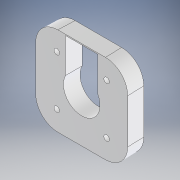
# Autodesk Inventor part: AA035
Saved by Autodesk Inventor 2017 SP1 (Build 210196100, 196)
## iProperties
Created: 2017-10-23
Part Number: AA035
Material: ABS Plastic
Document SubType Name: Modeling
Designer: Zach
Categories: <?xml version="1.0" encoding="UTF-16"?> <MemberInstance><Categories><FamilyTemplate><FamilyTemplateParameter ValueType="xs:double" Id="1" ObjectReferenceKey="da_z" ObjectType="kUserParameterObject"/><FamilyTemplateParameter ValueType="xs:double" Id="2" ObjectReferenceKey="da_b" ObjectType="kUserParameterObject"/><FamilyTemplateParameter ValueType="xs:double" Id="3" ObjectReferenceKey="da_beta" ObjectType="kUserParameterObject"/><FamilyTemplateParameter ValueType="xs:double" Id="4" ObjectReferenceKey="da_da" ObjectType="kUserParameterObject"/><FamilyTemplateParameter ValueType="xs:double" Id="5" ObjectReferenceKey="da_aw" ObjectType="kUserParameterObject"/><FamilyTemplateParameter ValueType="xs:string" Id="6" ObjectReferenceKey="EAIAABAAAACIAQAAAAAAAIAAAAAAAAAA" ObjectType="83910656" SubObjectId="SurfaceGeometry"/></FamilyTemplate><ParamToTemplateMap><ParamToTemplate CategoryParameter="//CategoryParameter[@InternalName='046C89C9-8512-4d59-83FE-43B91F4F132A']" TemplateParameter="1"/><ParamToTemplate CategoryParameter="//CategoryParameter[@InternalName='2552DF32-E462-4b46-AEBF-C6C7768E72AC']" TemplateParameter="2"/><ParamToTemplate CategoryParameter="//CategoryParameter[@InternalName='C9EE641D-15FC-4fae-A226-E94C4372FDD7']" TemplateParameter="3"/><ParamToTemplate><ParamToTemplate CategoryParameter="//CategoryParameter[@InternalName='00B6519A-459B-49c7-AD84-2E56D39A5744']" ConstantValue="0.341447"/></ParamToTemplate><ParamToTemplate><ParamToTemplate CategoryParameter="//CategoryParameter[@InternalName='04B31F0E-C7A6-4894-AA32-9629BEFACF47']" ConstantValue="1.000000"/></ParamToTemplate><ParamToTemplate><ParamToTemplate CategoryParameter="//CategoryParameter[@InternalName='43CBEC2E-7847-49e7-A936-2F7889FCB2D9']" ConstantValue="0.250000"/></ParamToTemplate><ParamToTemplate><ParamToTemplate CategoryParameter="//CategoryParameter[@InternalName='B1EFC894-105D-4ebd-86BF-FA20ED196853']" ConstantValue="0.350000"/></ParamToTemplate><ParamToTemplate><ParamToTemplate CategoryParameter="//CategoryParameter[@InternalName='51175063-3D10-4879-93E8-6246FE8B403D']" ConstantValue="2060000000.000000"/></ParamToTemplate><ParamToTemplate><ParamToTemplate CategoryParameter="//CategoryParameter[@InternalName='A3A52E27-4454-46a9-B0BD-C932399B70AF']" ConstantValue="0.300000"/></ParamToTemplate><ParamToTemplate><ParamToTemplate CategoryParameter="//CategoryParameter[@InternalName='91B76062-C214-41d9-B1B9-14D2AB99603D']" ConstantValue="0.200000"/></ParamToTemplate><ParamToTemplate><ParamToTemplate CategoryParameter="//CategoryParameter[@InternalName='374E806E-8B8A-4dda-A9AA-1039D6500AD2']" ConstantValue="5.000000"/></ParamToTemplate><ParamToTemplate><ParamToTemplate CategoryParameter="//CategoryParameter[@InternalName='2D373A89-B862-43d6-8D0B-0CBF12AB9F6C']" ConstantValue="0.392699"/></ParamToTemplate><ParamToTemplate CategoryParameter="//CategoryParameter[@InternalName='37777632-D6A2-4fac-9D53-DB8ACD95C989']" TemplateParameter="4"/><ParamToTemplate CategoryParameter="//CategoryParameter[@InternalName='FD1017F1-B727-4f7e-9707-0F86F1FF9423']" TemplateParameter="5"/><ParamToTemplate><ParamToTemplate CategoryParameter="//CategoryParameter[@InternalName='9E1B4470-B2D3-4ff1-B813-535BB4CDF51A']" ConstantValue="3520000.000000"/></ParamToTemplate><ParamToTemplate><ParamToTemplate CategoryParameter="//CategoryParameter[@InternalName='F8452263-BFF6-458c-9FB1-07C4B99E95CD']" ConstantValue="11400000.000000"/></ParamToTemplate><ParamToTemplate><ParamToTemplate CategoryParameter="//CategoryParameter[@InternalName='3E3BB259-FD49-497f-8171-6EBC954A3479']" ConstantValue="2.000000"/></ParamToTemplate><ParamToTemplate CategoryParameter="//CategoryParameter[@InternalName='27C3BAF2-7550-4e4b-AE2C-0DB134B7D9B7']" TemplateParameter="6"/></ParamToTemplateMap><Category DisplayName="Gear" InternalName="DC85795E-93AB-48d5-8EEE-5A27447B64BD" Mnemonic="Gear"><CategoryParameter DisplayName="z" InternalName="046C89C9-8512-4d59-83FE-43B91F4F132A" Mnemonic="z"/><CategoryParameter DisplayName="b" InternalName="2552DF32-E462-4b46-AEBF-C6C7768E72AC" Mnemonic="b"/><CategoryParameter DisplayName="||b|" InternalName="C9EE641D-15FC-4fae-A226-E94C4372FDD7" Mnemonic="beta"/><CategoryParameter DisplayName="x" InternalName="00B6519A-459B-49c7-AD84-2E56D39A5744" Mnemonic="x"/><CategoryParameter DisplayName="a*" InternalName="04B31F0E-C7A6-4894-AA32-9629BEFACF47" Mnemonic="a"/><CategoryParameter DisplayName="c*" InternalName="43CBEC2E-7847-49e7-A936-2F7889FCB2D9" Mnemonic="c"/><CategoryParameter DisplayName="r|.f|*" InternalName="B1EFC894-105D-4ebd-86BF-FA20ED196853" Mnemonic="rf"/><CategoryParameter DisplayName="E" InternalName="51175063-3D10-4879-93E8-6246FE8B403D" Mnemonic="E"/><CategoryParameter DisplayName="||m|" InternalName="A3A52E27-4454-46a9-B0BD-C932399B70AF" Mnemonic="mi"/><Category DisplayName="SpurGear" InternalName="26C5A22E-A91E-4dfd-A3B3-23CCAFAE1764" Mnemonic="SpurGear"><CategoryParameter DisplayName="m" InternalName="91B76062-C214-41d9-B1B9-14D2AB99603D" Mnemonic="m"/><CategoryParameter DisplayName="P" InternalName="374E806E-8B8A-4dda-A9AA-1039D6500AD2" Mnemonic="PP"/><CategoryParameter DisplayName="||a|" InternalName="2D373A89-B862-43d6-8D0B-0CBF12AB9F6C" Mnemonic="alpha"/><CategoryParameter DisplayName="d|.a|" InternalName="37777632-D6A2-4fac-9D53-DB8ACD95C989" Mnemonic="da"/><CategoryParameter DisplayName="a|.w|" InternalName="FD1017F1-B727-4f7e-9707-0F86F1FF9423" Mnemonic="aw"/><CategoryParameter DisplayName="||s||.Flim|" InternalName="9E1B4470-B2D3-4ff1-B813-535BB4CDF51A" Mnemonic="sFlim"/><CategoryParameter DisplayName="||s||.Hlim|" InternalName="F8452263-BFF6-458c-9FB1-07C4B99E95CD" Mnemonic="sHlim"/><CategoryParameter DisplayName="type" InternalName="3E3BB259-FD49-497f-8171-6EBC954A3479" Mnemonic="type"/><CategoryParameter DisplayName="PitchDiameter" InternalName="27C3BAF2-7550-4e4b-AE2C-0DB134B7D9B7" Mnemonic="IDS_PITCHDIAM"/></Category></Category></Categories></MemberInstance>
Density: 1.06 g/cm^3
Appearance: CR White
CustomPartVersion: 1
Author: Zach
Autodesk Inventor part; units mm, degrees
ref_plane "YZ Plane" through (0, 0, 0) normal (1, 0, 0) x (0, 1, 0)
ref_plane "XZ Plane" through (0, 0, 0) normal (0, 1, 0) x (-1, 0, 0)
ref_plane "XY Plane" through (0, 0, 0) normal (0, 0, 1) x (1, 0, 0)
sketch "Sketch3" plane through (0, 0, 0) normal (0, 0, 1) x (1, 0, 0)
  circle A0 centre (0, 0) radius 60
  dimension "d49" = 120
  constraints: 1 centre point, 1 coincident
  measures "d49" diameter of A0
extrude "Extrusion2" add sketch "Sketch3" along normal blind 67
sketch "Sketch4" plane through (0, 0, 0) normal (0, 0, -1) x (-1, 0, 0)
  circle A0 centre (0, 0) radius 4.25
  dimension "d52" = 8.5
  constraints: 1 centre point, 1 coincident
  measures "d52" diameter of A0
extrude "Extrusion3" cut sketch "Sketch4" against normal through all
ref_plane "Work Plane11" through (0, 0, 46) normal (0, 0, 1) x (1, 0, 0)
sketch "Sketch6" plane through (0, 0, 46) normal (0, 0, 1) x (1, 0, 0)
  line L0 (-27.5, -53.3268) -> (27.5, -53.3268)
  line L1 (27.5, -53.3268) -> (27.5, -61.3268)
  line L2 (27.5, -61.3268) -> (-27.5, -61.3268)
  line L3 (-27.5, -61.3268) -> (-27.5, -53.3268)
  circle A0 centre (0, 0) radius 4.25 construction
  circle A1 centre (0, 0) radius 60 construction
  dimension "d63" = 55
  dimension "d64" = 8
  constraints: 8 end point, 2 parallel, 2 point on circle, 1 horizontal, 1 perpendicular
  measures "d63" distance of L1.end L2.end
  measures "d64" distance of L0.end L1.end
extrude "Extrusion5" add sketch "Sketch6" along normal mid plane 42
sketch "Sketch7" plane through (0, 0, 46) normal (0, 0, 1) x (1, 0, 0)
  line L0 (-41, -61.3268) -> (41, -61.3268)
  line L1 (41.5215, -76.3268) -> (-41.5215, -76.3268)
  line L2 (27.5, -61.3268) -> (-27.5, -61.3268) projected
  line L3 (-41.5215, -76.3268) -> (-41, -61.3268)
  line L4 (41.5215, -76.3268) -> (41, -61.3268)
  point P0 (0, 0)
  point P1 (0, -61.3268)
  point P2 (0, -76.3268)
  dimension "d67" = 83.043
  dimension "d99" = 82
  dimension "d100" = 15
  constraints: 8 end point, 3 midpoint, 1 horizontal, 1 parallel, 1 vertical alignment
  measures "d67" distance of L1.start L1.end
  measures "d99" distance of L0.start L0.end
  measures "d100" distance between parallel lines of L0 L1
extrude "Extrusion6" add sketch "Sketch7" along normal mid plane 80
sketch "Sketch8" plane through (-41.5215, -76.3268, 86) normal (0, -1, 0) x (1, 0, 0)
  line L0 (64.0215, -62.5) -> (19.0215, -62.5) construction
  line L1 (19.0215, -62.5) -> (19.0215, -17.5) construction
  line L2 (19.0215, -17.5) -> (64.0215, -17.5) construction
  line L3 (64.0215, -17.5) -> (64.0215, -62.5) construction
  circle A0 centre (64.0215, -62.5) radius 2.5
  circle A1 centre (64.0215, -17.5) radius 2.5
  circle A2 centre (19.0215, -62.5) radius 2.5
  circle A3 centre (19.0215, -17.5) radius 2.5
  line L4 (0, 0) -> (83.043, 0) projected
  line L5 (83.043, 0) -> (83.043, -80) projected
  point P0 (23.25, -86)
  point P1 (41.5215, -17.5)
  point P2 (41.5215, 0)
  point P3 (64.0215, -40)
  point P4 (83.043, -40)
  dimension "d75" = 45
  dimension "d78" = 5
  dimension "d79" = 5
  dimension "d101" = 45
  dimension "d102" = 5
  dimension "d103" = 5
  constraints: 8 end point, 4 centre point, 4 coincident, 4 midpoint, 2 parallel, 1 horizontal, 1 horizontal alignment, 1 perpendicular, 1 vertical alignment
  measures "d75" distance of L0.end L1.end
  measures "d78" diameter of A2
  measures "d79" diameter of A3
  measures "d101" distance of L1.end L2.end
  measures "d102" diameter of A1
  measures "d103" diameter of A0
extrude "Extrusion7" cut sketch "Sketch8" against normal blind 25
sketch "Sketch9" plane through (-41.5215, -76.3268, 86) normal (0, -1, 0) x (1, 0, 0)
  circle A0 centre (41.5215, -40) radius 16.5
  circle A1 centre (19.0215, -62.5) radius 2.5 construction
  circle A2 centre (64.0215, -62.5) radius 2.5 construction
  circle A3 centre (64.0215, -17.5) radius 2.5 construction
  circle A4 centre (19.0215, -17.5) radius 2.5 construction
  line L0 (83.043, 0) -> (83.043, -80) construction
  line L1 (0, 0) -> (83.043, 0) construction
  line L2 (0, 0) -> (0, -80) construction
  line L3 (83.043, -80) -> (0, -80) construction
  point P0 (23.25, -86)
  point P1 (0, -40)
  point P2 (41.5215, 0)
  dimension "d82" = 33
  constraints: 2 midpoint, 1 centre point, 1 horizontal alignment, 1 vertical alignment
  measures "d82" diameter of A0
extrude "Extrusion8" cut sketch "Sketch9" against normal blind 45
sketch "Sketch14" plane through (0, 0, 46) normal (0, 0, 1) x (1, 0, 0)
  line L0 (16.5, -76.3268) -> (16.5, -31.3268) projected
  line L1 (16.5, -31.3268) -> (-16.5, -31.3268)
  line L2 (-16.5, -31.3268) -> (-16.5, -16.3268)
  line L3 (-16.5, -16.3268) -> (16.5, -16.3268)
  line L4 (16.5, -16.3268) -> (16.5, -31.3268)
  point P0 (0, 0)
  dimension "d91" = 33
  dimension "d92" = 15
  constraints: 8 end point, 2 parallel, 1 horizontal, 1 perpendicular
  measures "d91" distance of L2.end L3.end
  measures "d92" distance of L1.end L2.end
extrude "Extrusion10" cut sketch "Sketch14" along normal mid plane 33
sketch "Sketch15" plane through (16.5, -31.3268, 29.5) normal (-1, 0, 0) x (0, 0, 1)
  line L0 (33, 15) -> (0, 15) projected
  line L1 (0, 15) -> (0, 0) projected
  line L2 (0, 0) -> (16.5, 0) projected
  line L3 (16.5, 0) -> (33, 0) projected
  line L4 (33, 0) -> (33, 15) projected
  line L5 (24, 14) -> (9, 14)
  line L6 (9, 14) -> (9, 1)
  line L7 (9, 1) -> (24, 1)
  line L8 (24, 1) -> (24, 14)
  point P0 (-29.5, 31.3268)
  point P1 (16.5, 1)
  point P2 (24, 7.5)
  point P3 (33, 7.5)
  dimension "d95" = 15
  dimension "d96" = 13
  constraints: 8 end point, 3 midpoint, 2 parallel, 1 horizontal, 1 horizontal alignment, 1 perpendicular, 1 vertical alignment
  measures "d95" distance of L7.end L6.end
  measures "d96" distance of L6.end L5.end
extrude "Extrusion11" cut sketch "Sketch15" along normal through all contours L8 L7 L6 L5
fillet "Fillet4" radius 20 4 edges at (41.2608, -68.8268, 86) (41.2608, -68.8268, 6) (-41.2608, -68.8268, 86) (-41.2608, -68.8268, 6)
ref_plane "Work Plane15" through (0, 0, 25) normal (0, 0, -1) x (-0.9685832, -0.2486899, 0)
sketch "Sketch16" plane through (0, 0, 25) normal (0, 0, -1) x (-0.9685832, -0.2486899, 0)
  circle A0 centre (0, 0) radius 60
  circle A1 centre (0, 0) radius 63
  dimension "d107" = 3
  constraints: 2 centre point
  measures "d107" radial gap between concentric circles of A0 A1
extrude "Extrusion12" cut sketch "Sketch16" along normal through all contours A0 | A1
sketch "Sketch17" plane through (0, 0, 25) normal (0, 0, -1) x (-1, 0, 0)
  circle A0 centre (33.9004, 8.7041) radius 2.5
  circle A1 centre (9.4122, 33.7107) radius 2.5
  circle A2 centre (-24.4882, 25.0065) radius 2.5
  circle A3 centre (-33.9004, -8.7041) radius 2.5
  circle A4 centre (-9.4122, -33.7107) radius 2.5
  circle A5 centre (24.4882, -25.0065) radius 2.5
  line L0 (33.9004, 8.7041) -> (-33.9004, -8.7041) construction
  line L1 (-1.7981, -79.488) -> (39.8693, -68.7896)
  point P0 (0, 0)
  dimension "d108" = 5
  dimension "d109" = 35
  dimension "d112" = 360
  constraints: 6 centre point, 4 end point, 1 parallel, 13 other
  measures "d108" diameter of A0
  measures "d109" distance of point (0, 0) L0.start
extrude "Extrusion13" cut sketch "Sketch17" against normal blind 25 contours A0 | A1 | A2 | A3
sketch "Sketch20" plane through (0, 0, 67) normal (0, 0, 1) x (1, 0, 0)
  arc A0 (27.5, -53.3268) -> (-27.5, -53.3268) centre (0, 0) ccw projected
  circle A1 centre (0, 0) radius 60
  circle A2 centre (0, 0) radius 4.25 projected
  constraints: 1 coincident, 3 other
extrude "Extrusion15" add sketch "Sketch20" along normal blind 25
sketch "Sketch21" plane through (-21.5094, -76.3268, 6) normal (0, -1, 0) x (1, 0, 0)
  line L0 (36.0094, 79) -> (7.0094, 79)
  line L1 (7.0094, 79) -> (7.0094, 55)
  line L2 (7.0094, 55) -> (36.0094, 55)
  line L3 (36.0094, 55) -> (36.0094, 79)
  circle A0 centre (21.5094, 40) radius 16.5 projected
  line L4 (36.0094, 67) -> (7.0094, 67)
  point P0 (21.5094, -6)
  point P1 (21.5094, 67)
  dimension "d124" = 29
  dimension "d125" = 24
  dimension "d126" = 27
  constraints: 10 end point, 3 midpoint, 2 parallel, 1 horizontal, 1 perpendicular, 1 vertical alignment
  measures "d124" distance of L2.end L1.end
  measures "d125" distance of L1.end L0.end
  measures "d126" distance from line of L4 A0.centre
extrude "Extrusion16" cut sketch "Sketch21" against normal blind 15 contours L3 L4 L1 L0 | L3 L2 A0 L1 L4 | L2 A0 picked at (22.682, 55.3735)
sketch "Sketch22" plane through (-27.5, -61.3268, 67) normal (0, 1, 0) x (1, 0, 0)
  line L0 (55, 0) -> (55, 42) projected
  line L1 (0, 0) -> (0, 42) projected
  line L2 (0, 0) -> (3, 0)
  line L3 (55, 0) -> (55, -17.9115)
  line L4 (0, 0) -> (0, -17.9115)
  line L5 (5.9906, -19) -> (6.5121, -19) construction
  line L6 (-13.5, 1) -> (-14.0215, 1) construction
  circle A0 centre (5, -1.5) radius 2.5 projected
  line L7 (42, -18) -> (42, 6) projected
  line L8 (13, -18) -> (42, -18) projected
  line L9 (13, 6) -> (13, -18) projected
  line L10 (7, 0) -> (13, 0)
  line L11 (13, 0) -> (13, -18)
  line L12 (13, -18) -> (42, -18)
  line L13 (55, 0) -> (52, 0)
  circle A1 centre (50, -1.5) radius 2.5 projected
  line L14 (48, 0) -> (42, 0)
  line L15 (42, 0) -> (42, -18)
  arc A2 (48, 0) -> (52, 0) centre (50, -1.5) ccw
  arc A3 (3, 0) -> (7, 0) centre (5, -1.5) ccw
  line L16 (5.9906, -19) -> (6.2858, -19) projected
  line L17 (-13.5, 1) -> (-14.0215, 1) projected
  line L18 (5.9906, -19) -> (6.5121, -19) projected
  line L19 (48.4879, -19) -> (49.0094, -19) projected
  arc A4 (0, -17.9115) -> (6.2858, -19) centre (6.5121, 1) ccw
  arc A5 (48.4879, -19) -> (55, -17.9115) centre (48.488, 1.023) ccw
  line L20 (48.4879, -19) -> (6.2858, -19)
  line L21 (5.9906, -19) -> (49.0094, -19) projected
  ellipse E0 centre (5.9906, 1) end of major axis (-14.0215, 1) minor radius 20 (-14.0215, 1) -> (5.9906, -19) ccw projected
  line L22 (5.9906, -19) -> (6.5121, -19) projected
  ellipse E1 centre (6.5121, 1) end of major axis (-13.5, 1) minor radius 20 (-13.5, 1) -> (6.5121, -19) ccw projected
  line L23 (-13.5, 1) -> (-14.0215, 1) projected
  ellipse E2 centre (48.4879, 1) end of major axis (68.5, 1) minor radius 20 (48.4879, -19) -> (68.5, 1) ccw projected
  line L24 (48.4879, -19) -> (49.0094, -19) projected
  ellipse E3 centre (49.0094, 1) end of major axis (69.0215, 1) minor radius 20 (49.0094, -19) -> (69.0215, 1) ccw projected
  line L25 (69.0215, 1) -> (68.5, 1) projected
  point P0 (27.5, 67)
  point P1 (51.7891, -18.726)
  constraints: 22 end point, 11 point on circle, 4 centre point, 4 point on line, 3 perpendicular, 2 coincident, 2 collinear, 2 vertical, 1 horizontal, 1 horizontal alignment, 10 other
extrude "Extrusion17" add sketch "Sketch22" along normal blind 15 contours L2 A0 L10 L9 L8 L7 L14 A1 L13 L3 A5 L20 L18 A4 L4
sketch "Sketch23" plane through (-21.5094, -76.3268, 6) normal (0, -1, 0) x (1, 0, 0)
  line L0 (36.0094, 79) -> (36.0094, 55) projected
  line L1 (36.0094, 55) -> (7.0094, 55) projected
  line L2 (7.0094, 55) -> (7.0094, 79) projected
  line L3 (7.0094, 79) -> (36.0094, 79) projected
  point P0 (21.5094, -6)
extrude "Extrusion18" cut sketch "Sketch23" against normal blind 20
sketch "Sketch25" plane through (-21.5094, -56.3268, 6) normal (0, -1, 0) x (1, 0, 0)
  line L0 (36.0094, 55) -> (28.3833, 55) projected
  arc A0 (21.5094, 56.5) -> (5.0094, 40) centre (21.5094, 40) ccw projected
  line L1 (36.0094, 55) -> (7.0094, 55)
  line L2 (7.0094, 55) -> (7.0094, 47.874)
  line L3 (7.0094, 47.874) -> (36.0094, 47.874)
  line L4 (36.0094, 47.874) -> (36.0094, 55)
  point P0 (21.5094, -6)
  constraints: 8 end point, 2 parallel, 1 horizontal, 1 perpendicular, 1 point on circle, 1 vertical alignment
extrude "Extrusion20" cut sketch "Sketch25" along normal blind 25
sketch "Sketch26" plane through (0, 0, 92) normal (0, 0, 1) x (1, 0, 0)
  circle A0 centre (0, 0) radius 4.25 projected
  circle A1 centre (0, 0) radius 13.5
  dimension "d138" = 27
  constraints: 1 centre point, 1 coincident
  measures "d138" diameter of A1
extrude "Extrusion21" cut sketch "Sketch26" against normal blind 10
sketch "Sketch27" plane through (0, 0, 82) normal (0, 0, 1) x (1, 0, 0)
  circle A0 centre (9.525, 0) radius 1.5
  circle A1 centre (4.7625, 8.2489) radius 1.5
  circle A2 centre (-4.7625, 8.2489) radius 1.5
  circle A3 centre (-9.525, 0) radius 1.5
  circle A4 centre (-4.7625, -8.2489) radius 1.5
  circle A5 centre (4.7625, -8.2489) radius 1.5
  point P0 (0, 0)
  dimension "d141" = 3
  dimension "d142" = 9.525
  dimension "d145" = 360
  constraints: 6 centre point, 1 horizontal alignment, 13 other
  measures "d141" diameter of A0
  measures "d142" distance of point (0, 0) A0.centre
extrude "Extrusion22" cut sketch "Sketch27" against normal blind 15
sketch "Sketch28" plane through (0, 0, 0) normal (0, 1, 0) x (-1, 0, 0)
  circle A0 centre (0, 79.65) radius 1.5
  circle A1 centre (0, 84.75) radius 1.5
  line L0 (4.25, 82) -> (-4.25, 82) projected
  line L1 (0, 82) -> (0, 83.25)
  line L2 (0, 83.25) -> (0, 81.15)
  point P0 (0, 0)
  point P1 (0, 86.25)
  dimension "d151" = 3
  dimension "d150" = 3
  dimension "d153" = 1.25
  dimension "d166" = 2.1
  constraints: 4 end point, 4 vertical alignment, 2 point on circle, 2 vertical, 1 centre point, 1 midpoint, 2 other
  measures "d150" diameter of A1
  measures "d153" distance of L1.start L1.end
  measures "d166" distance of L1.end L2.end
extrude "Extrusion23" cut sketch "Sketch28" along normal through all
sketch "Sketch29" plane through (0, 0, 92) normal (0, 0, 1) x (1, 0, 0)
  circle A0 centre (0, 0) radius 17.5
  circle A1 centre (0, 0) radius 50
  dimension "d156" = 35
  dimension "d157" = 100
  constraints: 2 centre point, 2 coincident
  measures "d156" diameter of A0
  measures "d157" diameter of A1
extrude "Extrusion24" cut sketch "Sketch29" against normal blind 20
sketch "Sketch30" plane through (0, 0, 82) normal (0, 0, 1) x (1, 0, 0)
  circle A0 centre (0, 0) radius 17.5 projected
extrude "Extrusion25" cut sketch "Sketch30" along normal through all
sketch "Sketch32" plane through (0, 0, 82) normal (0, 0, 1) x (1, 0, 0)
  circle A0 centre (0, 0) radius 7.5
  dimension "d162" = 15
  constraints: 1 centre point, 1 coincident
  measures "d162" diameter of A0
extrude "Extrusion26" cut sketch "Sketch32" against normal blind 5
sketch "Sketch34" plane through (0, 0, 72) normal (0, 0, 1) x (1, 0, 0)
  line L0 (-14.5, -56.3268) -> (-14.5, -76.3268) projected
  line L1 (-14.5, -56.3268) -> (14.5, -56.3268)
  line L2 (14.5, -56.3268) -> (14.5, -21.3268)
  line L3 (14.5, -21.3268) -> (-14.5, -21.3268)
  line L4 (-14.5, -21.3268) -> (-14.5, -56.3268)
  line L5 (14.5, -76.3268) -> (14.5, -56.3268) projected
  point P0 (0, 0)
  dimension "d167" = 35
  constraints: 8 end point, 2 parallel, 1 coincident, 1 horizontal, 1 perpendicular
  measures "d167" distance of L1.end L2.end
extrude "Extrusion27" cut sketch "Sketch34" along normal blind 13 and the other way blind 20
sketch "Sketch35" plane through (-22.5, -61.3268, 23.5) normal (0, 1, 0) x (1, 0, 0)
  line L0 (-57.9857, -108.6859) -> (95.2212, -108.6859)
  line L1 (95.2212, -108.6859) -> (95.2212, 61.565)
  line L2 (95.2212, 61.565) -> (-57.9857, 61.565)
  line L3 (-57.9857, 61.565) -> (-57.9857, -108.6859)
  point P0 (22.5, 23.5)
  constraints: 8 end point, 2 parallel, 1 horizontal, 1 perpendicular
extrude "Extrusion28" cut sketch "Sketch35" along normal through all
equation "\"d43\" = da_aw"
equation "\"d46\" = da_aw"
equation "\"da_aw\" = 81.5"
body "Solid1"
